Autodesk Inventor part; units mm, degrees
(part 3 of 5)
  spline S592 degree 2 poles (-19.6244, -0.8792) (-19.506, -0.8792) (-19.3116, -0.7771) (-19.2273, -0.7009) knots 0 0 0 1 2 2 2
  line L506 (-17.4412, -1.0705) -> (-17.694, -1.0705)
  line L507 (-17.694, -1.0705) -> (-17.694, -0.2147)
  spline S593 degree 2 poles (-17.694, -0.2147) (-17.694, -0.111) (-17.7135, 0.0673) (-17.7427, 0.1208) knots 0 0 0 1 2 2 2
  spline S594 degree 2 poles (-17.7427, 0.1208) (-17.7735, 0.1775) (-17.8837, 0.2326) (-17.9777, 0.2326) knots 0 0 0 1 2 2 2
  spline S595 degree 2 poles (-17.9777, 0.2326) (-18.0717, 0.2326) (-18.271, 0.1321) (-18.3667, 0.0511) knots 0 0 0 1 2 2 2
  line L508 (-18.3667, 0.0511) -> (-18.3667, -1.0705)
  line L509 (-18.3667, -1.0705) -> (-18.6195, -1.0705)
  line L510 (-18.6195, -1.0705) -> (-18.6195, 0.4304)
  line L511 (-18.6195, 0.4304) -> (-18.3667, 0.4304)
  line L512 (-18.3667, 0.4304) -> (-18.3667, 0.2634)
  spline S596 degree 2 poles (-18.3667, 0.2634) (-18.2532, 0.3655) (-18.0344, 0.4725) (-17.9112, 0.4725) knots 0 0 0 1 2 2 2
  spline S597 degree 2 poles (-17.9112, 0.4725) (-17.6908, 0.4725) (-17.4412, 0.1808) (-17.4412, -0.0964) knots 0 0 0 1 2 2 2
  line L513 (-17.4412, -0.0964) -> (-17.4412, -1.0705)
  spline S598 degree 2 poles (-15.8529, -0.3201) (-15.8529, -0.6993) (-16.2175, -1.1126) (-16.5222, -1.1126) knots 0 0 0 1 2 2 2
  spline S599 degree 2 poles (-16.5222, -1.1126) (-16.8351, -1.1126) (-17.1932, -0.6863) (-17.1932, -0.3201) knots 0 0 0 1 2 2 2
  spline S600 degree 2 poles (-17.1932, -0.3201) (-17.1932, 0.056) (-16.8237, 0.4725) (-16.5222, 0.4725) knots 0 0 0 1 2 2 2
  spline S601 degree 2 poles (-16.5222, 0.4725) (-16.2175, 0.4725) (-15.8529, 0.0576) (-15.8529, -0.3201) knots 0 0 0 1 2 2 2
  spline S602 degree 2 poles (-16.1138, -0.3201) (-16.1138, -0.0283) (-16.3261, 0.2553) (-16.5222, 0.2553) knots 0 0 0 1 2 2 2
  spline S603 degree 2 poles (-16.5222, 0.2553) (-16.7184, 0.2553) (-16.9323, -0.0283) (-16.9323, -0.3201) knots 0 0 0 1 2 2 2
  spline S604 degree 2 poles (-16.9323, -0.3201) (-16.9323, -0.6037) (-16.7184, -0.8954) (-16.5222, -0.8954) knots 0 0 0 1 2 2 2
  spline S605 degree 2 poles (-16.5222, -0.8954) (-16.3278, -0.8954) (-16.1138, -0.6085) (-16.1138, -0.3201) knots 0 0 0 1 2 2 2
  line L514 (-14.7151, -1.0705) -> (-14.7151, 0.9295)
  line L515 (-14.7151, 0.9295) -> (-13.4639, 0.9295)
  line L516 (-13.4639, 0.9295) -> (-13.4639, 0.6929)
  line L517 (-13.4639, 0.6929) -> (-14.4493, 0.6929)
  line L518 (-14.4493, 0.6929) -> (-14.4493, 0.1451)
  line L519 (-14.4493, 0.1451) -> (-13.5304, 0.1451)
  line L520 (-13.5304, 0.1451) -> (-13.5304, -0.0915)
  line L521 (-13.5304, -0.0915) -> (-14.4493, -0.0915)
  line L522 (-14.4493, -0.0915) -> (-14.4493, -0.8338)
  line L523 (-14.4493, -0.8338) -> (-13.4639, -0.8338)
  line L524 (-13.4639, -0.8338) -> (-13.4639, -1.0705)
  line L525 (-13.4639, -1.0705) -> (-14.7151, -1.0705)
  line L526 (-11.4898, -1.0705) -> (-11.4898, -0.2017)
  spline S606 degree 2 poles (-11.4898, -0.2017) (-11.4898, -0.098) (-11.506, 0.0787) (-11.532, 0.1273) knots 0 0 0 1 2 2 2
  spline S607 degree 2 poles (-11.532, 0.1273) (-11.5579, 0.1808) (-11.6568, 0.2326) (-11.7427, 0.2326) knots 0 0 0 1 2 2 2
  spline S608 degree 2 poles (-11.7427, 0.2326) (-11.8205, 0.2326) (-11.9987, 0.137) (-12.0928, 0.0462) knots 0 0 0 1 2 2 2
  spline S609 degree 2 poles (-12.0928, 0.0462) (-12.0911, 0.0235) (-12.0879, -0.0397) (-12.0879, -0.0818) knots 0 0 0 1 2 2 2
  line L527 (-12.0879, -0.0818) -> (-12.0879, -1.0705)
  line L528 (-12.0879, -1.0705) -> (-12.3407, -1.0705)
  line L529 (-12.3407, -1.0705) -> (-12.3407, -0.2017)
  spline S610 degree 2 poles (-12.3407, -0.2017) (-12.3407, -0.098) (-12.3569, 0.0787) (-12.3829, 0.1273) knots 0 0 0 1 2 2 2
  spline S611 degree 2 poles (-12.3829, 0.1273) (-12.4088, 0.1808) (-12.5077, 0.2326) (-12.5936, 0.2326) knots 0 0 0 1 2 2 2
  spline S612 degree 2 poles (-12.5936, 0.2326) (-12.6746, 0.2326) (-12.8545, 0.1305) (-12.9388, 0.0511) knots 0 0 0 1 2 2 2
  line L530 (-12.9388, 0.0511) -> (-12.9388, -1.0705)
  line L531 (-12.9388, -1.0705) -> (-13.1916, -1.0705)
  line L532 (-13.1916, -1.0705) -> (-13.1916, 0.4304)
  line L533 (-13.1916, 0.4304) -> (-12.9388, 0.4304)
  line L534 (-12.9388, 0.4304) -> (-12.9388, 0.265)
  spline S613 degree 2 poles (-12.9388, 0.265) (-12.8399, 0.3639) (-12.6454, 0.4725) (-12.5287, 0.4725) knots 0 0 0 1 2 2 2
  spline S614 degree 2 poles (-12.5287, 0.4725) (-12.3958, 0.4725) (-12.19, 0.3509) (-12.1365, 0.2132) knots 0 0 0 1 2 2 2
  spline S615 degree 2 poles (-12.1365, 0.2132) (-12.0214, 0.3412) (-11.8043, 0.4725) (-11.6778, 0.4725) knots 0 0 0 1 2 2 2
  spline S616 degree 2 poles (-11.6778, 0.4725) (-11.5806, 0.4725) (-11.4218, 0.4125) (-11.3634, 0.3445) knots 0 0 0 1 2 2 2
  spline S617 degree 2 poles (-11.3634, 0.3445) (-11.3034, 0.2764) (-11.237, 0.0722) (-11.237, -0.0818) knots 0 0 0 1 2 2 2
  line L535 (-11.237, -0.0818) -> (-11.237, -1.0705)
  line L536 (-11.237, -1.0705) -> (-11.4898, -1.0705)
  spline S618 degree 2 poles (-10.0458, -0.9116) (-10.0765, -0.9343) (-10.1803, -1.0154) (-10.2289, -1.0397) knots 0 0 0 1 2 2 2
  spline S619 degree 2 poles (-10.2289, -1.0397) (-10.2953, -1.0753) (-10.4201, -1.1126) (-10.5336, -1.1126) knots 0 0 0 1 2 2 2
  spline S620 degree 2 poles (-10.5336, -1.1126) (-10.626, -1.1126) (-10.7929, -1.0429) (-10.8561, -0.9797) knots 0 0 0 1 2 2 2
  spline S621 degree 2 poles (-10.8561, -0.9797) (-10.9161, -0.9181) (-10.989, -0.7366) (-10.989, -0.6361) knots 0 0 0 1 2 2 2
  spline S622 degree 2 poles (-10.989, -0.6361) (-10.989, -0.4805) (-10.8577, -0.2601) (-10.7151, -0.1969) knots 0 0 0 1 2 2 2
  spline S623 degree 2 poles (-10.7151, -0.1969) (-10.5887, -0.1385) (-10.2451, -0.0948) (-10.0458, -0.0834) knots 0 0 0 1 2 2 2
  line L537 (-10.0458, -0.0834) -> (-10.0458, -0.0348)
  spline S624 degree 2 poles (-10.0458, -0.0348) (-10.0458, 0.0527) (-10.0992, 0.1613) (-10.1479, 0.1921) knots 0 0 0 1 2 2 2
  spline S625 degree 2 poles (-10.1479, 0.1921) (-10.1965, 0.2229) (-10.3359, 0.2423) (-10.4104, 0.2423) knots 0 0 0 1 2 2 2
  spline S626 degree 2 poles (-10.4104, 0.2423) (-10.4979, 0.2423) (-10.7346, 0.1905) (-10.8529, 0.1402) knots 0 0 0 1 2 2 2
  line L538 (-10.8529, 0.1402) -> (-10.8675, 0.1402)
  line L539 (-10.8675, 0.1402) -> (-10.8675, 0.3979)
  spline S627 degree 2 poles (-10.8675, 0.3979) (-10.7978, 0.4174) (-10.5368, 0.466) (-10.4088, 0.466) knots 0 0 0 1 2 2 2
  spline S628 degree 2 poles (-10.4088, 0.466) (-10.2532, 0.466) (-10.0409, 0.4174) (-9.9566, 0.3542) knots 0 0 0 1 2 2 2
  spline S629 degree 2 poles (-9.9566, 0.3542) (-9.874, 0.2926) (-9.7929, 0.0965) (-9.7929, -0.0445) knots 0 0 0 1 2 2 2
  line L540 (-9.7929, -0.0445) -> (-9.7929, -1.0705)
  line L541 (-9.7929, -1.0705) -> (-10.0458, -1.0705)
  line L542 (-10.0458, -1.0705) -> (-10.0458, -0.9116)
  line L543 (-10.0458, -0.7009) -> (-10.0458, -0.2844)
  spline S630 degree 2 poles (-10.0458, -0.2844) (-10.1365, -0.2925) (-10.4104, -0.3201) (-10.4963, -0.346) knots 0 0 0 1 2 2 2
  spline S631 degree 2 poles (-10.4963, -0.346) (-10.5968, -0.3768) (-10.7281, -0.5048) (-10.7281, -0.6183) knots 0 0 0 1 2 2 2
  spline S632 degree 2 poles (-10.7281, -0.6183) (-10.7281, -0.7479) (-10.5822, -0.8792) (-10.4428, -0.8792) knots 0 0 0 1 2 2 2
  spline S633 degree 2 poles (-10.4428, -0.8792) (-10.3245, -0.8792) (-10.13, -0.7771) (-10.0458, -0.7009) knots 0 0 0 1 2 2 2
  line L544 (-8.2597, -1.0705) -> (-8.5125, -1.0705)
  line L545 (-8.5125, -1.0705) -> (-8.5125, -0.2147)
  spline S634 degree 2 poles (-8.5125, -0.2147) (-8.5125, -0.111) (-8.532, 0.0673) (-8.5611, 0.1208) knots 0 0 0 1 2 2 2
  spline S635 degree 2 poles (-8.5611, 0.1208) (-8.5919, 0.1775) (-8.7022, 0.2326) (-8.7962, 0.2326) knots 0 0 0 1 2 2 2
  spline S636 degree 2 poles (-8.7962, 0.2326) (-8.8902, 0.2326) (-9.0895, 0.1321) (-9.1851, 0.0511) knots 0 0 0 1 2 2 2
  line L546 (-9.1851, 0.0511) -> (-9.1851, -1.0705)
  line L547 (-9.1851, -1.0705) -> (-9.438, -1.0705)
  line L548 (-9.438, -1.0705) -> (-9.438, 0.4304)
  line L549 (-9.438, 0.4304) -> (-9.1851, 0.4304)
  line L550 (-9.1851, 0.4304) -> (-9.1851, 0.2634)
  spline S637 degree 2 poles (-9.1851, 0.2634) (-9.0717, 0.3655) (-8.8529, 0.4725) (-8.7297, 0.4725) knots 0 0 0 1 2 2 2
  spline S638 degree 2 poles (-8.7297, 0.4725) (-8.5093, 0.4725) (-8.2597, 0.1808) (-8.2597, -0.0964) knots 0 0 0 1 2 2 2
  line L551 (-8.2597, -0.0964) -> (-8.2597, -1.0705)
  line L552 (-6.7378, -1.0705) -> (-6.9906, -1.0705)
  line L553 (-6.9906, -1.0705) -> (-6.9906, -0.9051)
  spline S639 degree 2 poles (-6.9906, -0.9051) (-7.1073, -1.0072) (-7.3164, -1.1126) (-7.4461, -1.1126) knots 0 0 0 1 2 2 2
  spline S640 degree 2 poles (-7.4461, -1.1126) (-7.5433, -1.1126) (-7.7167, -1.0478) (-7.7799, -0.9781) knots 0 0 0 1 2 2 2
  spline S641 degree 2 poles (-7.7799, -0.9781) (-7.8448, -0.9084) (-7.9161, -0.6961) (-7.9161, -0.5437) knots 0 0 0 1 2 2 2
  line L554 (-7.9161, -0.5437) -> (-7.9161, 0.4304)
  line L555 (-7.9161, 0.4304) -> (-7.6633, 0.4304)
  line L556 (-7.6633, 0.4304) -> (-7.6633, -0.4254)
  spline S642 degree 2 poles (-7.6633, -0.4254) (-7.6633, -0.5453) (-7.6454, -0.7025) (-7.6146, -0.7609) knots 0 0 0 1 2 2 2
  spline S643 degree 2 poles (-7.6146, -0.7609) (-7.5838, -0.8192) (-7.4785, -0.8727) (-7.3796, -0.8727) knots 0 0 0 1 2 2 2
  spline S644 degree 2 poles (-7.3796, -0.8727) (-7.2872, -0.8727) (-7.0782, -0.7674) (-6.9906, -0.6912) knots 0 0 0 1 2 2 2
  line L557 (-6.9906, -0.6912) -> (-6.9906, 0.4304)
  line L558 (-6.9906, 0.4304) -> (-6.7378, 0.4304)
  line L559 (-6.7378, 0.4304) -> (-6.7378, -1.0705)
  spline S645 degree 2 poles (-5.72, -1.1045) (-6.0798, -1.1045) (-6.4752, -0.7009) (-6.4752, -0.3282) knots 0 0 0 1 2 2 2
  spline S646 degree 2 poles (-6.4752, -0.3282) (-6.4752, 0.0381) (-6.0911, 0.4725) (-5.7816, 0.4725) knots 0 0 0 1 2 2 2
  spline S647 degree 2 poles (-5.7816, 0.4725) (-5.6422, 0.4725) (-5.4266, 0.3915) (-5.3472, 0.3056) knots 0 0 0 1 2 2 2
  spline S648 degree 2 poles (-5.3472, 0.3056) (-5.2662, 0.2197) (-5.1803, -0.0283) (-5.1803, -0.2082) knots 0 0 0 1 2 2 2
  line L560 (-5.1803, -0.2082) -> (-5.1803, -0.346)
  line L561 (-5.1803, -0.346) -> (-6.2192, -0.346)
  spline S649 degree 2 poles (-6.2192, -0.346) (-6.2192, -0.6069) (-5.9566, -0.8841) (-5.7232, -0.8841) knots 0 0 0 1 2 2 2
  spline S650 degree 2 poles (-5.7232, -0.8841) (-5.6406, -0.8841) (-5.4801, -0.8468) (-5.4153, -0.8176) knots 0 0 0 1 2 2 2
  spline S651 degree 2 poles (-5.4153, -0.8176) (-5.3472, -0.7852) (-5.2532, -0.7285) (-5.2224, -0.7025) knots 0 0 0 1 2 2 2
  line L562 (-5.2224, -0.7025) -> (-5.2078, -0.7025)
  line L563 (-5.2078, -0.7025) -> (-5.2078, -0.9781)
  spline S652 degree 2 poles (-5.2078, -0.9781) (-5.2516, -0.9959) (-5.3845, -1.0478) (-5.4364, -1.0624) knots 0 0 0 1 2 2 2
  spline S653 degree 2 poles (-5.4364, -1.0624) (-5.5093, -1.0834) (-5.6292, -1.1045) (-5.72, -1.1045) knots 0 0 0 1 2 2 2
  spline S654 degree 2 poles (-5.4266, -0.1531) (-5.4299, -0.051) (-5.472, 0.0981) (-5.5125, 0.1483) knots 0 0 0 1 2 2 2
  spline S655 degree 2 poles (-5.5125, 0.1483) (-5.5563, 0.2051) (-5.694, 0.265) (-5.7962, 0.265) knots 0 0 0 1 2 2 2
  spline S656 degree 2 poles (-5.7962, 0.265) (-5.8966, 0.265) (-6.0376, 0.2051) (-6.096, 0.1467) knots 0 0 0 1 2 2 2
  spline S657 degree 2 poles (-6.096, 0.1467) (-6.1527, 0.0868) (-6.2111, -0.0575) (-6.2192, -0.1531) knots 0 0 0 1 2 2 2
  line L564 (-6.2192, -0.1531) -> (-5.4266, -0.1531)
  line L565 (-4.6665, -1.0705) -> (-4.9193, -1.0705)
  line L566 (-4.9193, -1.0705) -> (-4.9193, 1.0187)
  line L567 (-4.9193, 1.0187) -> (-4.6665, 1.0187)
  line L568 (-4.6665, 1.0187) -> (-4.6665, -1.0705)
  spline S658 degree 2 poles (-3.6438, -1.1045) (-4.0036, -1.1045) (-4.3991, -0.7009) (-4.3991, -0.3282) knots 0 0 0 1 2 2 2
  spline S659 degree 2 poles (-4.3991, -0.3282) (-4.3991, 0.0381) (-4.015, 0.4725) (-3.7054, 0.4725) knots 0 0 0 1 2 2 2
  spline S660 degree 2 poles (-3.7054, 0.4725) (-3.566, 0.4725) (-3.3505, 0.3915) (-3.271, 0.3056) knots 0 0 0 1 2 2 2
  spline S661 degree 2 poles (-3.271, 0.3056) (-3.19, 0.2197) (-3.1041, -0.0283) (-3.1041, -0.2082) knots 0 0 0 1 2 2 2
  line L569 (-3.1041, -0.2082) -> (-3.1041, -0.346)
  line L570 (-3.1041, -0.346) -> (-4.143, -0.346)
  spline S662 degree 2 poles (-4.143, -0.346) (-4.143, -0.6069) (-3.8804, -0.8841) (-3.647, -0.8841) knots 0 0 0 1 2 2 2
  spline S663 degree 2 poles (-3.647, -0.8841) (-3.5644, -0.8841) (-3.4039, -0.8468) (-3.3391, -0.8176) knots 0 0 0 1 2 2 2
  spline S664 degree 2 poles (-3.3391, -0.8176) (-3.271, -0.7852) (-3.177, -0.7285) (-3.1462, -0.7025) knots 0 0 0 1 2 2 2
  line L571 (-3.1462, -0.7025) -> (-3.1317, -0.7025)
  line L572 (-3.1317, -0.7025) -> (-3.1317, -0.9781)
  spline S665 degree 2 poles (-3.1317, -0.9781) (-3.1754, -0.9959) (-3.3083, -1.0478) (-3.3602, -1.0624) knots 0 0 0 1 2 2 2
  spline S666 degree 2 poles (-3.3602, -1.0624) (-3.4331, -1.0834) (-3.553, -1.1045) (-3.6438, -1.1045) knots 0 0 0 1 2 2 2
  spline S667 degree 2 poles (-3.3505, -0.1531) (-3.3537, -0.051) (-3.3958, 0.0981) (-3.4364, 0.1483) knots 0 0 0 1 2 2 2
  spline S668 degree 2 poles (-3.4364, 0.1483) (-3.4801, 0.2051) (-3.6179, 0.265) (-3.72, 0.265) knots 0 0 0 1 2 2 2
  spline S669 degree 2 poles (-3.72, 0.265) (-3.8205, 0.265) (-3.9615, 0.2051) (-4.0198, 0.1467) knots 0 0 0 1 2 2 2
  spline S670 degree 2 poles (-4.0198, 0.1467) (-4.0765, 0.0868) (-4.1349, -0.0575) (-4.143, -0.1531) knots 0 0 0 1 2 2 2
  line L573 (-4.143, -0.1531) -> (-3.3505, -0.1531)
  spline S671 degree 2 poles (-28.3034, -3.4752) (-28.3034, -3.6697) (-28.5822, -3.9469) (-28.7767, -3.9469) knots 0 0 0 1 2 2 2
  spline S672 degree 2 poles (-28.7767, -3.9469) (-28.9712, -3.9469) (-29.2483, -3.6697) (-29.2483, -3.4752) knots 0 0 0 1 2 2 2
  spline S673 degree 2 poles (-29.2483, -3.4752) (-29.2483, -3.2807) (-28.9712, -3.0036) (-28.7767, -3.0036) knots 0 0 0 1 2 2 2
  spline S674 degree 2 poles (-28.7767, -3.0036) (-28.5822, -3.0036) (-28.3034, -3.2807) (-28.3034, -3.4752) knots 0 0 0 1 2 2 2
  spline S675 degree 2 poles (-21.8415, -3.7491) (-21.8415, -3.8982) (-21.955, -4.1268) (-22.049, -4.2013) knots 0 0 0 1 2 2 2
  spline S676 degree 2 poles (-22.049, -4.2013) (-22.1624, -4.2888) (-22.4201, -4.3634) (-22.6244, -4.3634) knots 0 0 0 1 2 2 2
  line L574 (-22.6244, -4.3634) -> (-23.1981, -4.3634)
  line L575 (-23.1981, -4.3634) -> (-23.1981, -2.3634)
  line L576 (-23.1981, -2.3634) -> (-22.6681, -2.3634)
  spline S677 degree 2 poles (-22.6681, -2.3634) (-22.4542, -2.3634) (-22.2402, -2.391) (-22.143, -2.4444) knots 0 0 0 1 2 2 2
  spline S678 degree 2 poles (-22.143, -2.4444) (-22.0344, -2.5012) (-21.9355, -2.6876) (-21.9355, -2.814) knots 0 0 0 1 2 2 2
  spline S679 degree 2 poles (-21.9355, -2.814) (-21.9355, -2.955) (-22.0846, -3.1786) (-22.2159, -3.2418) knots 0 0 0 1 2 2 2
  line L577 (-22.2159, -3.2418) -> (-22.2159, -3.2516)
  spline S680 degree 2 poles (-22.2159, -3.2516) (-22.0376, -3.3002) (-21.8415, -3.5579) (-21.8415, -3.7491) knots 0 0 0 1 2 2 2
  spline S681 degree 2 poles (-22.1187, -3.7605) (-22.1187, -3.647) (-22.1835, -3.5012) (-22.2808, -3.4493) knots 0 0 0 1 2 2 2
  spline S682 degree 2 poles (-22.2808, -3.4493) (-22.344, -3.4169) (-22.4931, -3.3974) (-22.6308, -3.3974) knots 0 0 0 1 2 2 2
  line L578 (-22.6308, -3.3974) -> (-22.9323, -3.3974)
  line L579 (-22.9323, -3.3974) -> (-22.9323, -4.1365)
  line L580 (-22.9323, -4.1365) -> (-22.7167, -4.1365)
  spline S683 degree 2 poles (-22.7167, -4.1365) (-22.5417, -4.1365) (-22.3407, -4.1041) (-22.2629, -4.0522) knots 0 0 0 1 2 2 2
  spline S684 degree 2 poles (-22.2629, -4.0522) (-22.1884, -3.9987) (-22.1187, -3.8658) (-22.1187, -3.7605) knots 0 0 0 1 2 2 2
  spline S685 degree 2 poles (-22.2127, -2.8512) (-22.2127, -2.7799) (-22.2613, -2.673) (-22.3148, -2.6422) knots 0 0 0 1 2 2 2
  spline S686 degree 2 poles (-22.3148, -2.6422) (-22.3796, -2.6065) (-22.5368, -2.5903) (-22.6778, -2.5903) knots 0 0 0 1 2 2 2
  line L581 (-22.6778, -2.5903) -> (-22.9323, -2.5903)
  line L582 (-22.9323, -2.5903) -> (-22.9323, -3.1754)
  line L583 (-22.9323, -3.1754) -> (-22.6308, -3.1754)
  spline S687 degree 2 poles (-22.6308, -3.1754) (-22.506, -3.1754) (-22.3877, -3.1495) (-22.3245, -3.1089) knots 0 0 0 1 2 2 2
  spline S688 degree 2 poles (-22.3245, -3.1089) (-22.2629, -3.07) (-22.2127, -2.9453) (-22.2127, -2.8512) knots 0 0 0 1 2 2 2
  spline S689 degree 2 poles (-20.7605, -4.2046) (-20.7913, -4.2273) (-20.895, -4.3083) (-20.9436, -4.3326) knots 0 0 0 1 2 2 2
  spline S690 degree 2 poles (-20.9436, -4.3326) (-21.0101, -4.3683) (-21.1349, -4.4055) (-21.2483, -4.4055) knots 0 0 0 1 2 2 2
  spline S691 degree 2 poles (-21.2483, -4.4055) (-21.3407, -4.4055) (-21.5077, -4.3359) (-21.5709, -4.2726) knots 0 0 0 1 2 2 2
  spline S692 degree 2 poles (-21.5709, -4.2726) (-21.6308, -4.2111) (-21.7038, -4.0295) (-21.7038, -3.929) knots 0 0 0 1 2 2 2
  spline S693 degree 2 poles (-21.7038, -3.929) (-21.7038, -3.7735) (-21.5725, -3.553) (-21.4299, -3.4898) knots 0 0 0 1 2 2 2
  spline S694 degree 2 poles (-21.4299, -3.4898) (-21.3034, -3.4315) (-20.9599, -3.3877) (-20.7605, -3.3764) knots 0 0 0 1 2 2 2
  line L584 (-20.7605, -3.3764) -> (-20.7605, -3.3277)
  spline S695 degree 2 poles (-20.7605, -3.3277) (-20.7605, -3.2402) (-20.814, -3.1316) (-20.8626, -3.1008) knots 0 0 0 1 2 2 2
  spline S696 degree 2 poles (-20.8626, -3.1008) (-20.9112, -3.07) (-21.0506, -3.0506) (-21.1252, -3.0506) knots 0 0 0 1 2 2 2
  spline S697 degree 2 poles (-21.1252, -3.0506) (-21.2127, -3.0506) (-21.4493, -3.1025) (-21.5676, -3.1527) knots 0 0 0 1 2 2 2
  line L585 (-21.5676, -3.1527) -> (-21.5822, -3.1527)
  line L586 (-21.5822, -3.1527) -> (-21.5822, -2.895)
  spline S698 degree 2 poles (-21.5822, -2.895) (-21.5125, -2.8756) (-21.2516, -2.8269) (-21.1235, -2.8269) knots 0 0 0 1 2 2 2
  spline S699 degree 2 poles (-21.1235, -2.8269) (-20.968, -2.8269) (-20.7556, -2.8756) (-20.6714, -2.9388) knots 0 0 0 1 2 2 2
  spline S700 degree 2 poles (-20.6714, -2.9388) (-20.5887, -3.0004) (-20.5077, -3.1965) (-20.5077, -3.3375) knots 0 0 0 1 2 2 2
  line L587 (-20.5077, -3.3375) -> (-20.5077, -4.3634)
  line L588 (-20.5077, -4.3634) -> (-20.7605, -4.3634)
  line L589 (-20.7605, -4.3634) -> (-20.7605, -4.2046)
  line L590 (-20.7605, -3.9939) -> (-20.7605, -3.5773)
  spline S701 degree 2 poles (-20.7605, -3.5773) (-20.8513, -3.5854) (-21.1252, -3.613) (-21.2111, -3.6389) knots 0 0 0 1 2 2 2
  spline S702 degree 2 poles (-21.2111, -3.6389) (-21.3116, -3.6697) (-21.4428, -3.7978) (-21.4428, -3.9112) knots 0 0 0 1 2 2 2
  spline S703 degree 2 poles (-21.4428, -3.9112) (-21.4428, -4.0409) (-21.297, -4.1722) (-21.1576, -4.1722) knots 0 0 0 1 2 2 2
  spline S704 degree 2 poles (-21.1576, -4.1722) (-21.0393, -4.1722) (-20.8448, -4.07) (-20.7605, -3.9939) knots 0 0 0 1 2 2 2
  line L591 (-18.9987, -4.3634) -> (-19.2516, -4.3634)
  line L592 (-19.2516, -4.3634) -> (-19.2516, -4.2111)
  spline S705 degree 2 poles (-19.2516, -4.2111) (-19.3099, -4.2597) (-19.3958, -4.3245) (-19.4542, -4.3521) knots 0 0 0 1 2 2 2
  spline S706 degree 2 poles (-19.4542, -4.3521) (-19.5077, -4.378) (-19.6227, -4.4055) (-19.6989, -4.4055) knots 0 0 0 1 2 2 2
  spline S707 degree 2 poles (-19.6989, -4.4055) (-19.8221, -4.4055) (-20.0295, -4.3034) (-20.1025, -4.2046) knots 0 0 0 1 2 2 2
  spline S708 degree 2 poles (-20.1025, -4.2046) (-20.1754, -4.1057) (-20.2564, -3.814) (-20.2564, -3.6243) knots 0 0 0 1 2 2 2
  spline S709 degree 2 poles (-20.2564, -3.6243) (-20.2564, -3.4266) (-20.1543, -3.1381) (-20.0652, -3.0295) knots 0 0 0 1 2 2 2
  spline S710 degree 2 poles (-20.0652, -3.0295) (-19.9825, -2.9323) (-19.7508, -2.8205) (-19.6227, -2.8205) knots 0 0 0 1 2 2 2
  spline S711 degree 2 poles (-19.6227, -2.8205) (-19.5109, -2.8205) (-19.344, -2.8707) (-19.2516, -2.9226) knots 0 0 0 1 2 2 2
  line L593 (-19.2516, -2.9226) -> (-19.2516, -2.2743)
  line L594 (-19.2516, -2.2743) -> (-18.9987, -2.2743)
  line L595 (-18.9987, -2.2743) -> (-18.9987, -4.3634)
  line L596 (-19.2516, -3.9987) -> (-19.2516, -3.1316)
  spline S712 degree 2 poles (-19.2516, -3.1316) (-19.3456, -3.0863) (-19.4947, -3.0522) (-19.5806, -3.0522) knots 0 0 0 1 2 2 2
  spline S713 degree 2 poles (-19.5806, -3.0522) (-19.7751, -3.0522) (-19.9955, -3.344) (-19.9955, -3.6195) knots 0 0 0 1 2 2 2
  spline S714 degree 2 poles (-19.9955, -3.6195) (-19.9955, -3.8853) (-19.827, -4.1657) (-19.6406, -4.1657) knots 0 0 0 1 2 2 2
  spline S715 degree 2 poles (-19.6406, -4.1657) (-19.5417, -4.1657) (-19.3407, -4.0749) (-19.2516, -3.9987) knots 0 0 0 1 2 2 2
  spline S716 degree 2 poles (-17.7962, -4.2046) (-17.827, -4.2273) (-17.9307, -4.3083) (-17.9793, -4.3326) knots 0 0 0 1 2 2 2
  spline S717 degree 2 poles (-17.9793, -4.3326) (-18.0458, -4.3683) (-18.1705, -4.4055) (-18.284, -4.4055) knots 0 0 0 1 2 2 2
  spline S718 degree 2 poles (-18.284, -4.4055) (-18.3764, -4.4055) (-18.5433, -4.3359) (-18.6065, -4.2726) knots 0 0 0 1 2 2 2
  spline S719 degree 2 poles (-18.6065, -4.2726) (-18.6665, -4.2111) (-18.7394, -4.0295) (-18.7394, -3.929) knots 0 0 0 1 2 2 2
  spline S720 degree 2 poles (-18.7394, -3.929) (-18.7394, -3.7735) (-18.6081, -3.553) (-18.4655, -3.4898) knots 0 0 0 1 2 2 2
  spline S721 degree 2 poles (-18.4655, -3.4898) (-18.3391, -3.4315) (-17.9955, -3.3877) (-17.7962, -3.3764) knots 0 0 0 1 2 2 2
  line L597 (-17.7962, -3.3764) -> (-17.7962, -3.3277)
  spline S722 degree 2 poles (-17.7962, -3.3277) (-17.7962, -3.2402) (-17.8496, -3.1316) (-17.8983, -3.1008) knots 0 0 0 1 2 2 2
  spline S723 degree 2 poles (-17.8983, -3.1008) (-17.9469, -3.07) (-18.0863, -3.0506) (-18.1608, -3.0506) knots 0 0 0 1 2 2 2
  spline S724 degree 2 poles (-18.1608, -3.0506) (-18.2483, -3.0506) (-18.485, -3.1025) (-18.6033, -3.1527) knots 0 0 0 1 2 2 2
  line L598 (-18.6033, -3.1527) -> (-18.6179, -3.1527)
  line L599 (-18.6179, -3.1527) -> (-18.6179, -2.895)
  spline S725 degree 2 poles (-18.6179, -2.895) (-18.5482, -2.8756) (-18.2872, -2.8269) (-18.1592, -2.8269) knots 0 0 0 1 2 2 2
  spline S726 degree 2 poles (-18.1592, -2.8269) (-18.0036, -2.8269) (-17.7913, -2.8756) (-17.707, -2.9388) knots 0 0 0 1 2 2 2
  spline S727 degree 2 poles (-17.707, -2.9388) (-17.6244, -3.0004) (-17.5433, -3.1965) (-17.5433, -3.3375) knots 0 0 0 1 2 2 2
  line L600 (-17.5433, -3.3375) -> (-17.5433, -4.3634)
  line L601 (-17.5433, -4.3634) -> (-17.7962, -4.3634)
  line L602 (-17.7962, -4.3634) -> (-17.7962, -4.2046)
  line L603 (-17.7962, -3.9939) -> (-17.7962, -3.5773)
  spline S728 degree 2 poles (-17.7962, -3.5773) (-17.8869, -3.5854) (-18.1608, -3.613) (-18.2467, -3.6389) knots 0 0 0 1 2 2 2
  spline S729 degree 2 poles (-18.2467, -3.6389) (-18.3472, -3.6697) (-18.4785, -3.7978) (-18.4785, -3.9112) knots 0 0 0 1 2 2 2
  spline S730 degree 2 poles (-18.4785, -3.9112) (-18.4785, -4.0409) (-18.3326, -4.1722) (-18.1932, -4.1722) knots 0 0 0 1 2 2 2
  spline S731 degree 2 poles (-18.1932, -4.1722) (-18.0749, -4.1722) (-17.8804, -4.07) (-17.7962, -3.9939) knots 0 0 0 1 2 2 2
  line L604 (-16.9307, -4.3634) -> (-17.1835, -4.3634)
  line L605 (-17.1835, -4.3634) -> (-17.1835, -2.2743)
  line L606 (-17.1835, -2.2743) -> (-16.9307, -2.2743)
  line L607 (-16.9307, -2.2743) -> (-16.9307, -4.3634)
  spline S732 degree 2 poles (-15.7232, -4.2046) (-15.754, -4.2273) (-15.8577, -4.3083) (-15.9064, -4.3326) knots 0 0 0 1 2 2 2
  spline S733 degree 2 poles (-15.9064, -4.3326) (-15.9728, -4.3683) (-16.0976, -4.4055) (-16.2111, -4.4055) knots 0 0 0 1 2 2 2
  spline S734 degree 2 poles (-16.2111, -4.4055) (-16.3034, -4.4055) (-16.4704, -4.3359) (-16.5336, -4.2726) knots 0 0 0 1 2 2 2
  spline S735 degree 2 poles (-16.5336, -4.2726) (-16.5936, -4.2111) (-16.6665, -4.0295) (-16.6665, -3.929) knots 0 0 0 1 2 2 2
  spline S736 degree 2 poles (-16.6665, -3.929) (-16.6665, -3.7735) (-16.5352, -3.553) (-16.3926, -3.4898) knots 0 0 0 1 2 2 2
  spline S737 degree 2 poles (-16.3926, -3.4898) (-16.2662, -3.4315) (-15.9226, -3.3877) (-15.7232, -3.3764) knots 0 0 0 1 2 2 2
  line L608 (-15.7232, -3.3764) -> (-15.7232, -3.3277)
  spline S738 degree 2 poles (-15.7232, -3.3277) (-15.7232, -3.2402) (-15.7767, -3.1316) (-15.8253, -3.1008) knots 0 0 0 1 2 2 2
  spline S739 degree 2 poles (-15.8253, -3.1008) (-15.874, -3.07) (-16.0133, -3.0506) (-16.0879, -3.0506) knots 0 0 0 1 2 2 2
  spline S740 degree 2 poles (-16.0879, -3.0506) (-16.1754, -3.0506) (-16.412, -3.1025) (-16.5304, -3.1527) knots 0 0 0 1 2 2 2
  line L609 (-16.5304, -3.1527) -> (-16.5449, -3.1527)
  line L610 (-16.5449, -3.1527) -> (-16.5449, -2.895)
  spline S741 degree 2 poles (-16.5449, -2.895) (-16.4752, -2.8756) (-16.2143, -2.8269) (-16.0863, -2.8269) knots 0 0 0 1 2 2 2
  spline S742 degree 2 poles (-16.0863, -2.8269) (-15.9307, -2.8269) (-15.7184, -2.8756) (-15.6341, -2.9388) knots 0 0 0 1 2 2 2
  spline S743 degree 2 poles (-15.6341, -2.9388) (-15.5514, -3.0004) (-15.4704, -3.1965) (-15.4704, -3.3375) knots 0 0 0 1 2 2 2
  line L611 (-15.4704, -3.3375) -> (-15.4704, -4.3634)
  line L612 (-15.4704, -4.3634) -> (-15.7232, -4.3634)
  line L613 (-15.7232, -4.3634) -> (-15.7232, -4.2046)
  line L614 (-15.7232, -3.9939) -> (-15.7232, -3.5773)
  spline S744 degree 2 poles (-15.7232, -3.5773) (-15.814, -3.5854) (-16.0879, -3.613) (-16.1738, -3.6389) knots 0 0 0 1 2 2 2
  spline S745 degree 2 poles (-16.1738, -3.6389) (-16.2743, -3.6697) (-16.4056, -3.7978) (-16.4056, -3.9112) knots 0 0 0 1 2 2 2
  spline S746 degree 2 poles (-16.4056, -3.9112) (-16.4056, -4.0409) (-16.2597, -4.1722) (-16.1203, -4.1722) knots 0 0 0 1 2 2 2
  spline S747 degree 2 poles (-16.1203, -4.1722) (-16.002, -4.1722) (-15.8075, -4.07) (-15.7232, -3.9939) knots 0 0 0 1 2 2 2
  line L615 (-13.4137, -4.3634) -> (-13.4137, -3.4947)
  spline S748 degree 2 poles (-13.4137, -3.4947) (-13.4137, -3.391) (-13.4299, -3.2143) (-13.4558, -3.1657) knots 0 0 0 1 2 2 2
  spline S749 degree 2 poles (-13.4558, -3.1657) (-13.4817, -3.1122) (-13.5806, -3.0603) (-13.6665, -3.0603) knots 0 0 0 1 2 2 2
  spline S750 degree 2 poles (-13.6665, -3.0603) (-13.7443, -3.0603) (-13.9226, -3.1559) (-14.0166, -3.2467) knots 0 0 0 1 2 2 2
  spline S751 degree 2 poles (-14.0166, -3.2467) (-14.015, -3.2694) (-14.0117, -3.3326) (-14.0117, -3.3747) knots 0 0 0 1 2 2 2
  line L616 (-14.0117, -3.3747) -> (-14.0117, -4.3634)
  line L617 (-14.0117, -4.3634) -> (-14.2646, -4.3634)
  line L618 (-14.2646, -4.3634) -> (-14.2646, -3.4947)
  spline S752 degree 2 poles (-14.2646, -3.4947) (-14.2646, -3.391) (-14.2808, -3.2143) (-14.3067, -3.1657) knots 0 0 0 1 2 2 2
  spline S753 degree 2 poles (-14.3067, -3.1657) (-14.3326, -3.1122) (-14.4315, -3.0603) (-14.5174, -3.0603) knots 0 0 0 1 2 2 2
  spline S754 degree 2 poles (-14.5174, -3.0603) (-14.5984, -3.0603) (-14.7783, -3.1624) (-14.8626, -3.2418) knots 0 0 0 1 2 2 2
  line L619 (-14.8626, -3.2418) -> (-14.8626, -4.3634)
  line L620 (-14.8626, -4.3634) -> (-15.1154, -4.3634)
  line L621 (-15.1154, -4.3634) -> (-15.1154, -2.8626)
  line L622 (-15.1154, -2.8626) -> (-14.8626, -2.8626)
  line L623 (-14.8626, -2.8626) -> (-14.8626, -3.0279)
  spline S755 degree 2 poles (-14.8626, -3.0279) (-14.7637, -2.929) (-14.5693, -2.8205) (-14.4526, -2.8205) knots 0 0 0 1 2 2 2
  spline S756 degree 2 poles (-14.4526, -2.8205) (-14.3197, -2.8205) (-14.1138, -2.942) (-14.0603, -3.0798) knots 0 0 0 1 2 2 2
  spline S757 degree 2 poles (-14.0603, -3.0798) (-13.9453, -2.9517) (-13.7281, -2.8205) (-13.6017, -2.8205) knots 0 0 0 1 2 2 2
  spline S758 degree 2 poles (-13.6017, -2.8205) (-13.5044, -2.8205) (-13.3456, -2.8804) (-13.2872, -2.9485) knots 0 0 0 1 2 2 2
  spline S759 degree 2 poles (-13.2872, -2.9485) (-13.2273, -3.0166) (-13.1608, -3.2208) (-13.1608, -3.3747) knots 0 0 0 1 2 2 2
  line L624 (-13.1608, -3.3747) -> (-13.1608, -4.3634)
  line L625 (-13.1608, -4.3634) -> (-13.4137, -4.3634)
  spline S760 degree 2 poles (-12.1543, -4.3974) (-12.5141, -4.3974) (-12.9096, -3.9939) (-12.9096, -3.6211) knots 0 0 0 1 2 2 2
  spline S761 degree 2 poles (-12.9096, -3.6211) (-12.9096, -3.2548) (-12.5255, -2.8205) (-12.2159, -2.8205) knots 0 0 0 1 2 2 2
  spline S762 degree 2 poles (-12.2159, -2.8205) (-12.0765, -2.8205) (-11.861, -2.9015) (-11.7816, -2.9874) knots 0 0 0 1 2 2 2
  spline S763 degree 2 poles (-11.7816, -2.9874) (-11.7005, -3.0733) (-11.6146, -3.3213) (-11.6146, -3.5012) knots 0 0 0 1 2 2 2
  line L626 (-11.6146, -3.5012) -> (-11.6146, -3.6389)
  line L627 (-11.6146, -3.6389) -> (-12.6535, -3.6389)
  spline S764 degree 2 poles (-12.6535, -3.6389) (-12.6535, -3.8999) (-12.391, -4.177) (-12.1576, -4.177) knots 0 0 0 1 2 2 2
  spline S765 degree 2 poles (-12.1576, -4.177) (-12.0749, -4.177) (-11.9145, -4.1397) (-11.8496, -4.1106) knots 0 0 0 1 2 2 2
  spline S766 degree 2 poles (-11.8496, -4.1106) (-11.7816, -4.0782) (-11.6876, -4.0214) (-11.6568, -3.9955) knots 0 0 0 1 2 2 2
  line L628 (-11.6568, -3.9955) -> (-11.6422, -3.9955)
  line L629 (-11.6422, -3.9955) -> (-11.6422, -4.271)
  spline S767 degree 2 poles (-11.6422, -4.271) (-11.6859, -4.2888) (-11.8188, -4.3407) (-11.8707, -4.3553) knots 0 0 0 1 2 2 2
  spline S768 degree 2 poles (-11.8707, -4.3553) (-11.9436, -4.3764) (-12.0636, -4.3974) (-12.1543, -4.3974) knots 0 0 0 1 2 2 2
  spline S769 degree 2 poles (-11.861, -3.4461) (-11.8642, -3.344) (-11.9064, -3.1948) (-11.9469, -3.1446) knots 0 0 0 1 2 2 2
  spline S770 degree 2 poles (-11.9469, -3.1446) (-11.9906, -3.0879) (-12.1284, -3.0279) (-12.2305, -3.0279) knots 0 0 0 1 2 2 2
  spline S771 degree 2 poles (-12.2305, -3.0279) (-12.331, -3.0279) (-12.472, -3.0879) (-12.5304, -3.1462) knots 0 0 0 1 2 2 2
  spline S772 degree 2 poles (-12.5304, -3.1462) (-12.5871, -3.2062) (-12.6454, -3.3504) (-12.6535, -3.4461) knots 0 0 0 1 2 2 2
  line L630 (-12.6535, -3.4461) -> (-11.861, -3.4461)
  line L631 (-10.1803, -4.3634) -> (-10.4331, -4.3634)
  line L632 (-10.4331, -4.3634) -> (-10.4331, -3.5076)
  spline S773 degree 2 poles (-10.4331, -3.5076) (-10.4331, -3.4039) (-10.4526, -3.2256) (-10.4817, -3.1722) knots 0 0 0 1 2 2 2
  spline S774 degree 2 poles (-10.4817, -3.1722) (-10.5125, -3.1154) (-10.6227, -3.0603) (-10.7167, -3.0603) knots 0 0 0 1 2 2 2
  spline S775 degree 2 poles (-10.7167, -3.0603) (-10.8107, -3.0603) (-11.0101, -3.1608) (-11.1057, -3.2418) knots 0 0 0 1 2 2 2
  line L633 (-11.1057, -3.2418) -> (-11.1057, -4.3634)
  line L634 (-11.1057, -4.3634) -> (-11.3586, -4.3634)
  line L635 (-11.3586, -4.3634) -> (-11.3586, -2.8626)
  line L636 (-11.3586, -2.8626) -> (-11.1057, -2.8626)
  line L637 (-11.1057, -2.8626) -> (-11.1057, -3.0295)
  spline S776 degree 2 poles (-11.1057, -3.0295) (-10.9923, -2.9274) (-10.7735, -2.8205) (-10.6503, -2.8205) knots 0 0 0 1 2 2 2
  spline S777 degree 2 poles (-10.6503, -2.8205) (-10.4299, -2.8205) (-10.1803, -3.1122) (-10.1803, -3.3893) knots 0 0 0 1 2 2 2
  line L638 (-10.1803, -3.3893) -> (-10.1803, -4.3634)
  spline S778 degree 2 poles (-9.3715, -4.3926) (-9.5774, -4.3926) (-9.8091, -4.1576) (-9.8091, -3.9031) knots 0 0 0 1 2 2 2
  line L639 (-9.8091, -3.9031) -> (-9.8091, -3.0717)
  line L640 (-9.8091, -3.0717) -> (-9.9793, -3.0717)
  line L641 (-9.9793, -3.0717) -> (-9.9793, -2.8626)
  line L642 (-9.9793, -2.8626) -> (-9.8091, -2.8626)
  line L643 (-9.8091, -2.8626) -> (-9.8091, -2.4315)
  line L644 (-9.8091, -2.4315) -> (-9.5563, -2.4315)
  line L645 (-9.5563, -2.4315) -> (-9.5563, -2.8626)
  line L646 (-9.5563, -2.8626) -> (-9.0911, -2.8626)
  line L647 (-9.0911, -2.8626) -> (-9.0911, -3.0717)
  line L648 (-9.0911, -3.0717) -> (-9.5563, -3.0717)
  line L649 (-9.5563, -3.0717) -> (-9.5563, -3.7864)
  spline S779 degree 2 poles (-9.5563, -3.7864) (-9.5563, -3.8999) (-9.5482, -4.0247) (-9.5206, -4.0782) knots 0 0 0 1 2 2 2
  spline S780 degree 2 poles (-9.5206, -4.0782) (-9.4979, -4.1252) (-9.3958, -4.1722) (-9.3083, -4.1722) knots 0 0 0 1 2 2 2
  spline S781 degree 2 poles (-9.3083, -4.1722) (-9.2467, -4.1722) (-9.1317, -4.1349) (-9.1057, -4.1235) knots 0 0 0 1 2 2 2
  line L650 (-9.1057, -4.1235) -> (-9.0911, -4.1235)
  line L651 (-9.0911, -4.1235) -> (-9.0911, -4.3504)
  spline S782 degree 2 poles (-9.0911, -4.3504) (-9.1624, -4.3699) (-9.3083, -4.3926) (-9.3715, -4.3926) knots 0 0 0 1 2 2 2
  line L652 (-8.647, -4.3634) -> (-8.8999, -4.3634)
  line L653 (-8.8999, -4.3634) -> (-8.8999, -2.8626)
  line L654 (-8.8999, -2.8626) -> (-8.647, -2.8626)
  line L655 (-8.647, -2.8626) -> (-8.647, -4.3634)
  line L656 (-8.6292, -2.613) -> (-8.9161, -2.613)
  line L657 (-8.9161, -2.613) -> (-8.9161, -2.3504)
  line L658 (-8.9161, -2.3504) -> (-8.6292, -2.3504)
  line L659 (-8.6292, -2.3504) -> (-8.6292, -2.613)
  line L660 (-6.2013, -2.6) -> (-7.1317, -2.6)
  line L661 (-7.1317, -2.6) -> (-7.1317, -3.1641)
  line L662 (-7.1317, -3.1641) -> (-6.2402, -3.1641)
  line L663 (-6.2402, -3.1641) -> (-6.2402, -3.4007)
  line L664 (-6.2402, -3.4007) -> (-7.1317, -3.4007)
  line L665 (-7.1317, -3.4007) -> (-7.1317, -4.3634)
  line L666 (-7.1317, -4.3634) -> (-7.3975, -4.3634)
  line L667 (-7.3975, -4.3634) -> (-7.3975, -2.3634)
  line L668 (-7.3975, -2.3634) -> (-6.2013, -2.3634)
  line L669 (-6.2013, -2.3634) -> (-6.2013, -2.6)
  line L670 (-5.7248, -4.3634) -> (-5.9777, -4.3634)
  line L671 (-5.9777, -4.3634) -> (-5.9777, -2.8626)
  line L672 (-5.9777, -2.8626) -> (-5.7248, -2.8626)
  line L673 (-5.7248, -2.8626) -> (-5.7248, -4.3634)
  line L674 (-5.707, -2.613) -> (-5.9939, -2.613)
  line L675 (-5.9939, -2.613) -> (-5.9939, -2.3504)
  line L676 (-5.9939, -2.3504) -> (-5.707, -2.3504)
  line L677 (-5.707, -2.3504) -> (-5.707, -2.613)
  line L678 (-5.096, -4.3634) -> (-5.3488, -4.3634)
  line L679 (-5.3488, -4.3634) -> (-5.3488, -2.2743)
  line L680 (-5.3488, -2.2743) -> (-5.096, -2.2743)
  line L681 (-5.096, -2.2743) -> (-5.096, -4.3634)
  line L682 (-4.4671, -4.3634) -> (-4.72, -4.3634)
  line L683 (-4.72, -4.3634) -> (-4.72, -2.8626)
  line L684 (-4.72, -2.8626) -> (-4.4671, -2.8626)
  line L685 (-4.4671, -2.8626) -> (-4.4671, -4.3634)
  line L686 (-4.4493, -2.613) -> (-4.7362, -2.613)
  line L687 (-4.7362, -2.613) -> (-4.7362, -2.3504)
  line L688 (-4.7362, -2.3504) -> (-4.4493, -2.3504)
  line L689 (-4.4493, -2.3504) -> (-4.4493, -2.613)
  spline S783 degree 2 poles (-2.8383, -3.5725) (-2.8383, -3.9485) (-3.1965, -4.3926) (-3.4704, -4.3926) knots 0 0 0 1 2 2 2
  spline S784 degree 2 poles (-3.4704, -4.3926) (-3.5822, -4.3926) (-3.754, -4.3407) (-3.8432, -4.2872) knots 0 0 0 1 2 2 2
  line L690 (-3.8432, -4.2872) -> (-3.8432, -4.9161)
  line L691 (-3.8432, -4.9161) -> (-4.096, -4.9161)
  line L692 (-4.096, -4.9161) -> (-4.096, -2.8626)
  line L693 (-4.096, -2.8626) -> (-3.8432, -2.8626)
  line L694 (-3.8432, -2.8626) -> (-3.8432, -3.0198)
  spline S785 degree 2 poles (-3.8432, -3.0198) (-3.7492, -2.9339) (-3.519, -2.8205) (-3.3845, -2.8205) knots 0 0 0 1 2 2 2
  spline S786 degree 2 poles (-3.3845, -2.8205) (-3.1268, -2.8205) (-2.8383, -3.2289) (-2.8383, -3.5725) knots 0 0 0 1 2 2 2
  spline S787 degree 2 poles (-3.0992, -3.6017) (-3.0992, -3.344) (-3.2629, -3.0603) (-3.4461, -3.0603) knots 0 0 0 1 2 2 2
  spline S788 degree 2 poles (-3.4461, -3.0603) (-3.553, -3.0603) (-3.754, -3.1559) (-3.8432, -3.2305) knots 0 0 0 1 2 2 2
  line L695 (-3.8432, -3.2305) -> (-3.8432, -4.083)
  spline S789 degree 2 poles (-3.8432, -4.083) (-3.7443, -4.13) (-3.6033, -4.1657) (-3.5125, -4.1657) knots 0 0 0 1 2 2 2
  spline S790 degree 2 poles (-3.5125, -4.1657) (-3.3164, -4.1657) (-3.0992, -3.8772) (-3.0992, -3.6017) knots 0 0 0 1 2 2 2
  spline S791 degree 2 poles (-1.318, -3.5725) (-1.318, -3.9485) (-1.6762, -4.3926) (-1.9501, -4.3926) knots 0 0 0 1 2 2 2
  spline S792 degree 2 poles (-1.9501, -4.3926) (-2.062, -4.3926) (-2.2338, -4.3407) (-2.3229, -4.2872) knots 0 0 0 1 2 2 2
  line L696 (-2.3229, -4.2872) -> (-2.3229, -4.9161)
  line L697 (-2.3229, -4.9161) -> (-2.5757, -4.9161)
  line L698 (-2.5757, -4.9161) -> (-2.5757, -2.8626)
  line L699 (-2.5757, -2.8626) -> (-2.3229, -2.8626)
  line L700 (-2.3229, -2.8626) -> (-2.3229, -3.0198)
  spline S793 degree 2 poles (-2.3229, -3.0198) (-2.2289, -2.9339) (-1.9987, -2.8205) (-1.8642, -2.8205) knots 0 0 0 1 2 2 2
  spline S794 degree 2 poles (-1.8642, -2.8205) (-1.6065, -2.8205) (-1.318, -3.2289) (-1.318, -3.5725) knots 0 0 0 1 2 2 2
  spline S795 degree 2 poles (-1.579, -3.6017) (-1.579, -3.344) (-1.7427, -3.0603) (-1.9258, -3.0603) knots 0 0 0 1 2 2 2
  spline S796 degree 2 poles (-1.9258, -3.0603) (-2.0328, -3.0603) (-2.2338, -3.1559) (-2.3229, -3.2305) knots 0 0 0 1 2 2 2
  line L701 (-2.3229, -3.2305) -> (-2.3229, -4.083)
  spline S797 degree 2 poles (-2.3229, -4.083) (-2.224, -4.13) (-2.083, -4.1657) (-1.9923, -4.1657) knots 0 0 0 1 2 2 2
  spline S798 degree 2 poles (-1.9923, -4.1657) (-1.7962, -4.1657) (-1.579, -3.8772) (-1.579, -3.6017) knots 0 0 0 1 2 2 2
  spline S799 degree 2 poles (0.1779, -3.613) (0.1779, -3.9923) (-0.1868, -4.4055) (-0.4915, -4.4055) knots 0 0 0 1 2 2 2
  spline S800 degree 2 poles (-0.4915, -4.4055) (-0.8043, -4.4055) (-1.1624, -3.9793) (-1.1624, -3.613) knots 0 0 0 1 2 2 2
  spline S801 degree 2 poles (-1.1624, -3.613) (-1.1624, -3.237) (-0.7929, -2.8205) (-0.4915, -2.8205) knots 0 0 0 1 2 2 2
  spline S802 degree 2 poles (-0.4915, -2.8205) (-0.1868, -2.8205) (0.1779, -3.2354) (0.1779, -3.613) knots 0 0 0 1 2 2 2
  spline S803 degree 2 poles (-0.083, -3.613) (-0.083, -3.3213) (-0.2953, -3.0376) (-0.4915, -3.0376) knots 0 0 0 1 2 2 2
  spline S804 degree 2 poles (-0.4915, -3.0376) (-0.6876, -3.0376) (-0.9015, -3.3213) (-0.9015, -3.613) knots 0 0 0 1 2 2 2
  spline S805 degree 2 poles (-0.9015, -3.613) (-0.9015, -3.8966) (-0.6876, -4.1884) (-0.4915, -4.1884) knots 0 0 0 1 2 2 2
  spline S806 degree 2 poles (-0.4915, -4.1884) (-0.297, -4.1884) (-0.083, -3.9015) (-0.083, -3.613) knots 0 0 0 1 2 2 2
  spline S807 degree 2 poles (-28.3034, -6.7682) (-28.3034, -6.9627) (-28.5822, -7.2398) (-28.7767, -7.2398) knots 0 0 0 1 2 2 2
  spline S808 degree 2 poles (-28.7767, -7.2398) (-28.9712, -7.2398) (-29.2483, -6.9627) (-29.2483, -6.7682) knots 0 0 0 1 2 2 2
  spline S809 degree 2 poles (-29.2483, -6.7682) (-29.2483, -6.5737) (-28.9712, -6.2965) (-28.7767, -6.2965) knots 0 0 0 1 2 2 2
  spline S810 degree 2 poles (-28.7767, -6.2965) (-28.5822, -6.2965) (-28.3034, -6.5737) (-28.3034, -6.7682) knots 0 0 0 1 2 2 2
  line L702 (-21.7475, -5.6564) -> (-22.4364, -7.6564)
  line L703 (-22.4364, -7.6564) -> (-22.7232, -7.6564)
  line L704 (-22.7232, -7.6564) -> (-23.412, -5.6564)
  line L705 (-23.412, -5.6564) -> (-23.1268, -5.6564)
  line L706 (-23.1268, -5.6564) -> (-22.5725, -7.3176)
  line L707 (-22.5725, -7.3176) -> (-22.0182, -5.6564)
  line L708 (-22.0182, -5.6564) -> (-21.7475, -5.6564)
  line L709 (-21.318, -7.6564) -> (-21.5709, -7.6564)
  line L710 (-21.5709, -7.6564) -> (-21.5709, -6.1555)
  line L711 (-21.5709, -6.1555) -> (-21.318, -6.1555)
  line L712 (-21.318, -6.1555) -> (-21.318, -7.6564)
  line L713 (-21.3002, -5.9059) -> (-21.5871, -5.9059)
  line L714 (-21.5871, -5.9059) -> (-21.5871, -5.6434)
  line L715 (-21.5871, -5.6434) -> (-21.3002, -5.6434)
  line L716 (-21.3002, -5.6434) -> (-21.3002, -5.9059)
  spline S811 degree 2 poles (-20.4931, -7.6855) (-20.6989, -7.6855) (-20.9307, -7.4505) (-20.9307, -7.1961) knots 0 0 0 1 2 2 2
  line L717 (-20.9307, -7.1961) -> (-20.9307, -6.3646)
  line L718 (-20.9307, -6.3646) -> (-21.1009, -6.3646)
  line L719 (-21.1009, -6.3646) -> (-21.1009, -6.1555)
  line L720 (-21.1009, -6.1555) -> (-20.9307, -6.1555)
  line L721 (-20.9307, -6.1555) -> (-20.9307, -5.7244)
  line L722 (-20.9307, -5.7244) -> (-20.6778, -5.7244)
  line L723 (-20.6778, -5.7244) -> (-20.6778, -6.1555)
  line L724 (-20.6778, -6.1555) -> (-20.2127, -6.1555)
  line L725 (-20.2127, -6.1555) -> (-20.2127, -6.3646)
  line L726 (-20.2127, -6.3646) -> (-20.6778, -6.3646)
  line L727 (-20.6778, -6.3646) -> (-20.6778, -7.0794)
  spline S812 degree 2 poles (-20.6778, -7.0794) (-20.6778, -7.1928) (-20.6697, -7.3176) (-20.6422, -7.3711) knots 0 0 0 1 2 2 2
  spline S813 degree 2 poles (-20.6422, -7.3711) (-20.6195, -7.4181) (-20.5174, -7.4651) (-20.4299, -7.4651) knots 0 0 0 1 2 2 2
  spline S814 degree 2 poles (-20.4299, -7.4651) (-20.3683, -7.4651) (-20.2532, -7.4278) (-20.2273, -7.4165) knots 0 0 0 1 2 2 2
  line L728 (-20.2273, -7.4165) -> (-20.2127, -7.4165)
  line L729 (-20.2127, -7.4165) -> (-20.2127, -7.6434)
  spline S815 degree 2 poles (-20.2127, -7.6434) (-20.284, -7.6628) (-20.4299, -7.6855) (-20.4931, -7.6855) knots 0 0 0 1 2 2 2
  spline S816 degree 2 poles (-19.5725, -7.6855) (-19.7783, -7.6855) (-20.0101, -7.4505) (-20.0101, -7.1961) knots 0 0 0 1 2 2 2
  line L730 (-20.0101, -7.1961) -> (-20.0101, -6.3646)
  line L731 (-20.0101, -6.3646) -> (-20.1803, -6.3646)
  line L732 (-20.1803, -6.3646) -> (-20.1803, -6.1555)
  line L733 (-20.1803, -6.1555) -> (-20.0101, -6.1555)
  line L734 (-20.0101, -6.1555) -> (-20.0101, -5.7244)
  line L735 (-20.0101, -5.7244) -> (-19.7573, -5.7244)
  line L736 (-19.7573, -5.7244) -> (-19.7573, -6.1555)
  line L737 (-19.7573, -6.1555) -> (-19.2921, -6.1555)
  line L738 (-19.2921, -6.1555) -> (-19.2921, -6.3646)
  line L739 (-19.2921, -6.3646) -> (-19.7573, -6.3646)
  line L740 (-19.7573, -6.3646) -> (-19.7573, -7.0794)
  spline S817 degree 2 poles (-19.7573, -7.0794) (-19.7573, -7.1928) (-19.7492, -7.3176) (-19.7216, -7.3711) knots 0 0 0 1 2 2 2
  spline S818 degree 2 poles (-19.7216, -7.3711) (-19.6989, -7.4181) (-19.5968, -7.4651) (-19.5093, -7.4651) knots 0 0 0 1 2 2 2
  spline S819 degree 2 poles (-19.5093, -7.4651) (-19.4477, -7.4651) (-19.3326, -7.4278) (-19.3067, -7.4165) knots 0 0 0 1 2 2 2
  line L741 (-19.3067, -7.4165) -> (-19.2921, -7.4165)
  line L742 (-19.2921, -7.4165) -> (-19.2921, -7.6434)
  spline S820 degree 2 poles (-19.2921, -7.6434) (-19.3634, -7.6628) (-19.5093, -7.6855) (-19.5725, -7.6855) knots 0 0 0 1 2 2 2
  line L743 (-18.848, -7.6564) -> (-19.1009, -7.6564)
  line L744 (-19.1009, -7.6564) -> (-19.1009, -6.1555)
  line L745 (-19.1009, -6.1555) -> (-18.848, -6.1555)
  line L746 (-18.848, -6.1555) -> (-18.848, -7.6564)
  line L747 (-18.8302, -5.9059) -> (-19.1171, -5.9059)
  line L748 (-19.1171, -5.9059) -> (-19.1171, -5.6434)
  line L749 (-19.1171, -5.6434) -> (-18.8302, -5.6434)
  line L750 (-18.8302, -5.6434) -> (-18.8302, -5.9059)
  spline S821 degree 2 poles (-16.7605, -7.6952) (-16.9728, -7.6952) (-17.3245, -7.5656) (-17.4509, -7.4343) knots 0 0 0 1 2 2 2
  spline S822 degree 2 poles (-17.4509, -7.4343) (-17.5774, -7.3014) (-17.7119, -6.9092) (-17.7119, -6.6547) knots 0 0 0 1 2 2 2
  spline S823 degree 2 poles (-17.7119, -6.6547) (-17.7119, -6.4132) (-17.5757, -6.0307) (-17.4493, -5.8946) knots 0 0 0 1 2 2 2
  spline S824 degree 2 poles (-17.4493, -5.8946) (-17.3278, -5.7633) (-16.9712, -5.6207) (-16.7589, -5.6207) knots 0 0 0 1 2 2 2
  spline S825 degree 2 poles (-16.7589, -5.6207) (-16.6568, -5.6207) (-16.472, -5.6499) (-16.3877, -5.6758) knots 0 0 0 1 2 2 2
  spline S826 degree 2 poles (-16.3877, -5.6758) (-16.3197, -5.6952) (-16.1543, -5.7666) (-16.1041, -5.7925) knots 0 0 0 1 2 2 2
  line L751 (-16.1041, -5.7925) -> (-16.1041, -6.1134)
  line L752 (-16.1041, -6.1134) -> (-16.1268, -6.1134)
  spline S827 degree 2 poles (-16.1268, -6.1134) (-16.177, -6.0696) (-16.2824, -5.9902) (-16.3796, -5.9448) knots 0 0 0 1 2 2 2
  spline S828 degree 2 poles (-16.3796, -5.9448) (-16.4607, -5.9043) (-16.6697, -5.8508) (-16.7897, -5.8508) knots 0 0 0 1 2 2 2
  spline S829 degree 2 poles (-16.7897, -5.8508) (-17.0782, -5.8508) (-17.4347, -6.2852) (-17.4347, -6.6466) knots 0 0 0 1 2 2 2
  spline S830 degree 2 poles (-17.4347, -6.6466) (-17.4347, -6.8476) (-17.3407, -7.1491) (-17.2516, -7.2528) knots 0 0 0 1 2 2 2
  spline S831 degree 2 poles (-17.2516, -7.2528) (-17.1657, -7.3565) (-16.9226, -7.4651) (-16.7702, -7.4651) knots 0 0 0 1 2 2 2
  spline S832 degree 2 poles (-16.7702, -7.4651) (-16.6584, -7.4651) (-16.4347, -7.4327) (-16.3586, -7.4003) knots 0 0 0 1 2 2 2
  line L753 (-16.3586, -7.4003) -> (-16.3586, -6.8833)
  line L754 (-16.3586, -6.8833) -> (-16.8221, -6.8833)
  line L755 (-16.8221, -6.8833) -> (-16.8221, -6.6499)
  line L756 (-16.8221, -6.6499) -> (-16.096, -6.6499)
  line L757 (-16.096, -6.6499) -> (-16.096, -7.5234)
  spline S833 degree 2 poles (-16.096, -7.5234) (-16.1462, -7.5461) (-16.318, -7.6158) (-16.391, -7.6369) knots 0 0 0 1 2 2 2
  spline S834 degree 2 poles (-16.391, -7.6369) (-16.4898, -7.6661) (-16.6487, -7.6952) (-16.7605, -7.6952) knots 0 0 0 1 2 2 2
  spline S835 degree 2 poles (-14.9453, -7.4975) (-14.9761, -7.5202) (-15.0798, -7.6012) (-15.1284, -7.6256) knots 0 0 0 1 2 2 2
  spline S836 degree 2 poles (-15.1284, -7.6256) (-15.1949, -7.6612) (-15.3197, -7.6985) (-15.4331, -7.6985) knots 0 0 0 1 2 2 2
  spline S837 degree 2 poles (-15.4331, -7.6985) (-15.5255, -7.6985) (-15.6924, -7.6288) (-15.7556, -7.5656) knots 0 0 0 1 2 2 2
  spline S838 degree 2 poles (-15.7556, -7.5656) (-15.8156, -7.504) (-15.8885, -7.3225) (-15.8885, -7.222) knots 0 0 0 1 2 2 2
  spline S839 degree 2 poles (-15.8885, -7.222) (-15.8885, -7.0664) (-15.7573, -6.846) (-15.6146, -6.7828) knots 0 0 0 1 2 2 2
  spline S840 degree 2 poles (-15.6146, -6.7828) (-15.4882, -6.7244) (-15.1446, -6.6807) (-14.9453, -6.6693) knots 0 0 0 1 2 2 2
  line L758 (-14.9453, -6.6693) -> (-14.9453, -6.6207)
  spline S841 degree 2 poles (-14.9453, -6.6207) (-14.9453, -6.5332) (-14.9987, -6.4246) (-15.0474, -6.3938) knots 0 0 0 1 2 2 2
  spline S842 degree 2 poles (-15.0474, -6.3938) (-15.096, -6.363) (-15.2354, -6.3435) (-15.3099, -6.3435) knots 0 0 0 1 2 2 2
  spline S843 degree 2 poles (-15.3099, -6.3435) (-15.3975, -6.3435) (-15.6341, -6.3954) (-15.7524, -6.4457) knots 0 0 0 1 2 2 2
  line L759 (-15.7524, -6.4457) -> (-15.767, -6.4457)
  line L760 (-15.767, -6.4457) -> (-15.767, -6.188)
  spline S844 degree 2 poles (-15.767, -6.188) (-15.6973, -6.1685) (-15.4364, -6.1199) (-15.3083, -6.1199) knots 0 0 0 1 2 2 2
  spline S845 degree 2 poles (-15.3083, -6.1199) (-15.1527, -6.1199) (-14.9404, -6.1685) (-14.8561, -6.2317) knots 0 0 0 1 2 2 2
  spline S846 degree 2 poles (-14.8561, -6.2317) (-14.7735, -6.2933) (-14.6924, -6.4894) (-14.6924, -6.6304) knots 0 0 0 1 2 2 2
  line L761 (-14.6924, -6.6304) -> (-14.6924, -7.6564)
  line L762 (-14.6924, -7.6564) -> (-14.9453, -7.6564)
  line L763 (-14.9453, -7.6564) -> (-14.9453, -7.4975)
  line L764 (-14.9453, -7.2868) -> (-14.9453, -6.8703)
  spline S847 degree 2 poles (-14.9453, -6.8703) (-15.036, -6.8784) (-15.3099, -6.9059) (-15.3958, -6.9319) knots 0 0 0 1 2 2 2
  spline S848 degree 2 poles (-15.3958, -6.9319) (-15.4963, -6.9627) (-15.6276, -7.0907) (-15.6276, -7.2042) knots 0 0 0 1 2 2 2
  spline S849 degree 2 poles (-15.6276, -7.2042) (-15.6276, -7.3338) (-15.4817, -7.4651) (-15.3423, -7.4651) knots 0 0 0 1 2 2 2
  spline S850 degree 2 poles (-15.3423, -7.4651) (-15.224, -7.4651) (-15.0295, -7.363) (-14.9453, -7.2868) knots 0 0 0 1 2 2 2
  spline S851 degree 2 poles (-13.0798, -6.8816) (-13.0798, -7.2495) (-13.4364, -7.6985) (-13.7054, -7.6985) knots 0 0 0 1 2 2 2
  spline S852 degree 2 poles (-13.7054, -7.6985) (-13.827, -7.6985) (-14.0004, -7.6385) (-14.0846, -7.5867) knots 0 0 0 1 2 2 2
  line L765 (-14.0846, -7.5867) -> (-14.1009, -7.6564)
  line L766 (-14.1009, -7.6564) -> (-14.3375, -7.6564)
  line L767 (-14.3375, -7.6564) -> (-14.3375, -5.5672)
  line L768 (-14.3375, -5.5672) -> (-14.0846, -5.5672)
  line L769 (-14.0846, -5.5672) -> (-14.0846, -6.3128)
  spline S853 degree 2 poles (-14.0846, -6.3128) (-13.989, -6.2269) (-13.767, -6.1134) (-13.626, -6.1134) knots 0 0 0 1 2 2 2
  spline S854 degree 2 poles (-13.626, -6.1134) (-13.3715, -6.1134) (-13.0798, -6.5202) (-13.0798, -6.8816) knots 0 0 0 1 2 2 2
  spline S855 degree 2 poles (-13.3407, -6.9011) (-13.3407, -6.632) (-13.5044, -6.3533) (-13.6859, -6.3533) knots 0 0 0 1 2 2 2
  spline S856 degree 2 poles (-13.6859, -6.3533) (-13.7881, -6.3533) (-13.9987, -6.4505) (-14.0846, -6.5251) knots 0 0 0 1 2 2 2
  line L770 (-14.0846, -6.5251) -> (-14.0846, -7.3857)
  spline S857 degree 2 poles (-14.0846, -7.3857) (-13.989, -7.4327) (-13.8415, -7.4716) (-13.754, -7.4716) knots 0 0 0 1 2 2 2
  spline S858 degree 2 poles (-13.754, -7.4716) (-13.5611, -7.4716) (-13.3407, -7.1977) (-13.3407, -6.9011) knots 0 0 0 1 2 2 2
  line L771 (-12.0214, -6.4262) -> (-12.0344, -6.4262)
  spline S859 degree 2 poles (-12.0344, -6.4262) (-12.0636, -6.4181) (-12.1268, -6.4149) (-12.1705, -6.4149) knots 0 0 0 1 2 2 2
  spline S860 degree 2 poles (-12.1705, -6.4149) (-12.2727, -6.4149) (-12.4736, -6.504) (-12.5644, -6.5915) knots 0 0 0 1 2 2 2
  line L772 (-12.5644, -6.5915) -> (-12.5644, -7.6564)
  line L773 (-12.5644, -7.6564) -> (-12.8172, -7.6564)
  line L774 (-12.8172, -7.6564) -> (-12.8172, -6.1555)
  line L775 (-12.8172, -6.1555) -> (-12.5644, -6.1555)
  line L776 (-12.5644, -6.1555) -> (-12.5644, -6.3792)
  spline S861 degree 2 poles (-12.5644, -6.3792) (-12.4266, -6.256) (-12.2208, -6.1555) (-12.1235, -6.1555) knots 0 0 0 1 2 2 2
  spline S862 degree 2 poles (-12.1235, -6.1555) (-12.0846, -6.1555) (-12.0458, -6.1588) (-12.0214, -6.1636) knots 0 0 0 1 2 2 2
  line L777 (-12.0214, -6.1636) -> (-12.0214, -6.4262)
  line L778 (-11.5676, -7.6564) -> (-11.8205, -7.6564)
  line L779 (-11.8205, -7.6564) -> (-11.8205, -6.1555)
  line L780 (-11.8205, -6.1555) -> (-11.5676, -6.1555)
  line L781 (-11.5676, -6.1555) -> (-11.5676, -7.6564)
  line L782 (-11.5498, -5.9059) -> (-11.8367, -5.9059)
  line L783 (-11.8367, -5.9059) -> (-11.8367, -5.6434)
  line L784 (-11.8367, -5.6434) -> (-11.5498, -5.6434)
  line L785 (-11.5498, -5.6434) -> (-11.5498, -5.9059)
  spline S863 degree 2 poles (-10.5449, -7.6904) (-10.9047, -7.6904) (-11.3002, -7.2868) (-11.3002, -6.914) knots 0 0 0 1 2 2 2
  spline S864 degree 2 poles (-11.3002, -6.914) (-11.3002, -6.5478) (-10.9161, -6.1134) (-10.6065, -6.1134) knots 0 0 0 1 2 2 2
  spline S865 degree 2 poles (-10.6065, -6.1134) (-10.4671, -6.1134) (-10.2516, -6.1944) (-10.1722, -6.2803) knots 0 0 0 1 2 2 2
  spline S866 degree 2 poles (-10.1722, -6.2803) (-10.0911, -6.3662) (-10.0052, -6.6142) (-10.0052, -6.7941) knots 0 0 0 1 2 2 2